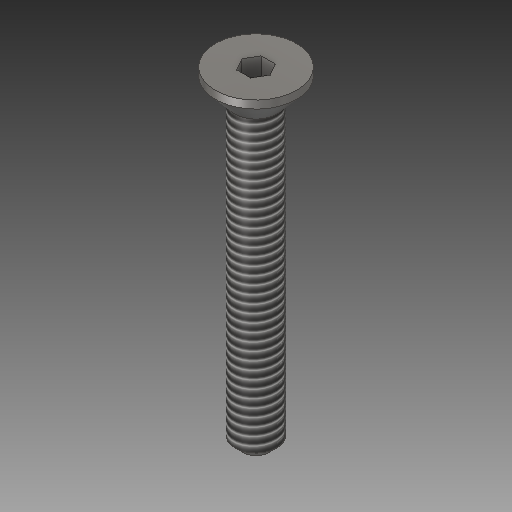
# Autodesk Inventor part: 8-32 UNC Flathead Bolt
Saved by Autodesk Inventor 2018 (Build 220112000, 112)
## iProperties
Created: 2018-01-08
Part Number: 8-32 UNC Flathead Bolt
Material: Stainless Steel
Document SubType Name: Modeling
Designer: 232963
Density: 8 g/cm^3
Appearance: Semi-Polished
Mass: 3.67809 g
Surface Area: 5.14876 cm^2
Volume: 0.459761 cm^3
Author: 232963
Autodesk Inventor part; units mm, degrees
ref_plane "YZ Plane" through (0, 0, 0) normal (1, 0, 0) x (0, 1, 0)
ref_plane "XZ Plane" through (0, 0, 0) normal (0, 1, 0) x (-1, 0, 0)
ref_plane "XY Plane" through (0, 0, 0) normal (0, 0, 1) x (1, 0, 0)
sketch "Sketch1" plane through (0, 0, 0) normal (0, 0, 1) x (1, 0, 0)
  line L0 (0, 0) -> (3.937, 0)
  line L1 (3.937, 0) -> (3.937, 31.75)
  line L2 (3.937, 31.75) -> (0, 31.75)
  line L3 (0, 31.75) -> (0, 0)
  line L4 (2.032, 28.7965) -> (2.032, 0)
  line L5 (2.032, 28.7965) -> (3.937, 30.988)
  dimension "d0" = 3.937
  dimension "d1" = 31.75
  dimension "d2" = 2.032
  dimension "d3" = 0.762
  dimension "d4" = 41
  constraints: 12 end point, 2 parallel, 2 perpendicular, 2 point on line, 1 horizontal
  measures "d0" distance of L2.end L1.end
  measures "d1" distance of L1.end L0.end
  measures "d2" distance between parallel lines of L3 L4
  measures "d3" distance of L1.end L5.end
  measures "d4" angle of L3 L5
revolve "Revolution1" add sketch "Sketch1" angle 360 about axis through (0, 31.75, 0) along (0, -1, 0) contours L3 L2 L1 L5 L4 L0
chamfer "Chamfer1" distance 0.762 angle 45 1 edges at (-2.032, 0, 0)
thread "Thread1" size "8-32 UNC" class "2A" standard "ANSI Unified Screw Threads" full length
sketch "Sketch2" plane through (0, 31.75, 0) normal (0, 1, 0) x (1, 0, 0)
  line L0 (1.3638, 0) -> (0.6819, -1.1811)
  line L1 (0.6819, -1.1811) -> (-0.6819, -1.1811)
  line L2 (-0.6819, -1.1811) -> (-1.3638, 0)
  line L3 (-1.3638, 0) -> (-0.6819, 1.1811)
  line L4 (-0.6819, 1.1811) -> (0.6819, 1.1811)
  line L5 (0.6819, 1.1811) -> (1.3638, 0)
  point P0 (0, 0)
  point P1 (0, 0)
  point P2 (0, 0)
  dimension "d11" = 2.3622
  constraints: 12 end point, 1 coincident, 13 other
  measures "d11" distance between parallel lines of L1 L4
extrude "Extrusion1" cut sketch "Sketch2" against normal blind 2.286
body "Solid1"
